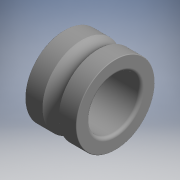
# Autodesk Inventor part: W 619/2.5 R_PART1
Saved by Autodesk Inventor 2017.3 (Build 213256000, 256)
## iProperties
Part Number: W 619/2.5 R_PART1
Material: Generic
Catalog Web Link: www.cadenas.de
Description: -Deep groove ball bearings
Vendor: SKF
Document SubType Name: Modeling
Designer: partserver
Manufacturer: SKF
Mass: 0.0157937 g
Surface Area: 0.623845 cm^2
Volume: 0.0157937 cm^3
Density: 1 g/cm^3
Appearance: PSOLRGB-175-175-175
Category: PARTsolutions
Company: SKF
Title: W 619/2.5 R_PART1
Author: Cadenas PARTsolutions
Comments: Deep groove ball bearings
PSOL_IDENT_0: {$CADENAS_DATA\23d-libs\skf\bearings_units_and_housings\ball_bearings\deep_groove_ball_bearings\bb1_
PSOL_IDENT_1: 001_101.prj},201 {VTYP=3D},{NB=W 619/2.5 R_PART1},{LINA=W 619/2.5 R_PART1},{NN=BB1_001_101_PART1},{N
PSOL_IDENT_2: OPRJ=TRUE},{DATE=19.12.2019 14:34:47},{GEOMDATE=18.12.2019 13:53:11},{VERSION=},{LINEID=21370},{WBVA
PSOL_IDENT_3: R=},{WBNUMERIC=}  {NB=W 619/2.5 R_PART1},{LINA=W 619/2.5 R_PART1},{KT=DUMMY},{PRODUCTID=},{DESIGNATI
PSOL_IDENT_4: ON=W 619/2.5 R},{DD=2.500},{D=7.000},{B=2.500},{C=0.700},{DD1=3.85},{DD2=0.00},{D1=5.65},{D2=0.00},{
PSOL_IDENT_5: D3=8.500},{D4=0.000},{HH=MIN},{BB=0.000},{FF=0.00},{R0MAX=MIN},{R0=MIN},{R12=0.15},{PITCH=4.75},{DW=
PSOL_IDENT_6: 1.200},{DDAMIN=3.300},{DDAMAX=MIN},{DDBMIN=MIN},{DDBMAX=MIN},{DBMIN=MIN},{DAMAX=MIN},{BBAMIN=MIN},{C
PSOL_IDENT_7: AMAX=MIN},{RAMAX=0.150},{LOAD1=0.221},{LOAD2=0.067},{LOAD3=0.003},{SPEED1=160000},{SPEED2=100000},{K
PSOL_IDENT_8: R=0.025},{F0=6.600},{Z=7},{II=1},{MASS=0.001},{BEARING=W 619/2.5 R},{RING=},{HELP=0.675},{HELP2=0.67
PSOL_IDENT_9: 5},{DD1ALG=1.925},{YALG=1.925},{PITCH1=4.750},{DW1=1.200},{YALG1=2.825},{HALG1=0.675},{SH=1.925},{CU=
PSOL_IDENT_10: 0.260},{DESIGN=dgbbw},{HALG=0.675},{B1=-1.215},{SHIELDHELP=1}
NB: W 619/2.5 R_PART1
NT: Deep groove ball bearings
NBSYN: $DESIGNATION._PART1
LINA: W 619/2.5 R_PART1
CATALOG: SKF
SUPPLIER: SKF
ARTICLENO: W 619/2.5 R_PART1
BOMINFO: W 619/2.5 R_PART1
CREATOR: CADENAS GmbH
Autodesk Inventor part; units mm, degrees
ref_plane "YZ Plane" through (0, 0, 0) normal (1, 0, 0) x (0, 1, 0)
ref_plane "XZ Plane" through (0, 0, 0) normal (0, 1, 0) x (-1, 0, 0)
ref_plane "XY Plane" through (0, 0, 0) normal (0, 0, 1) x (1, 0, 0)
sketch "Sketch_10" plane through (0, 0, 0) normal (0, 0, 1) x (1, 0, 0)
  line L0 (50, 0) -> (-50, 0)
  line L1 (0, 1.895) -> (0, 1.4)
  arc A0 (0, 1.4) -> (0.15, 1.25) centre (0.15, 1.4) ccw
  line L2 (0.15, 1.25) -> (2.35, 1.25)
  arc A1 (2.35, 1.25) -> (2.5, 1.4) centre (2.35, 1.4) ccw
  line L3 (2.5, 1.4) -> (2.5, 1.895)
  arc A2 (2.5, 1.895) -> (2.47, 1.925) centre (2.47, 1.895) ccw
  line L4 (2.47, 1.925) -> (1.6469, 1.925)
  arc A3 (0.8531, 1.925) -> (1.6469, 1.925) centre (1.25, 2.375) ccw
  line L5 (0.8531, 1.925) -> (0.03, 1.925)
  arc A4 (0.03, 1.925) -> (0, 1.895) centre (0.03, 1.895) ccw
  constraints: 12 end point, 10 point on circle, 5 centre point
revolve "Revolution1" add sketch "Sketch_10" angle 360 about axis through (50, 0, 0) along (1, 0, 0)
body "Solid1"
